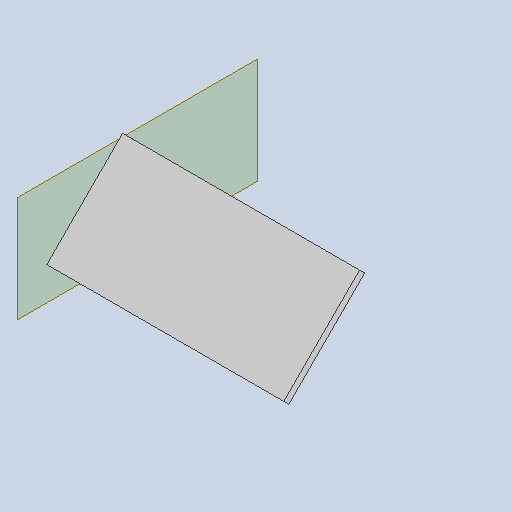
# Autodesk Inventor part: plugg
Saved by Autodesk Inventor 2022 (Build 260153000, 153)
## iProperties
Created: 2022-12-25
Part Number: plugg
Material: Generic
Document SubType Name: Modeling
Designer: Kamil
Density: 1 g/cm^3
Appearance: Default
Author: Kamil
Autodesk Inventor part; units mm, degrees
ref_plane "YZ Plane" through (0, 0, 0) normal (1, 0, 0) x (0, 1, 0)
ref_plane "XZ Plane" through (0, 0, 0) normal (0, 1, 0) x (-1, 0, 0)
ref_plane "Work Plane1" through (89.5496, -22.0458, 63.3377) normal (-1, 0, 0) x (0, -1, 0)
sketch "Sketch1" plane through (89.5496, -22.0458, 63.3377) normal (-1, 0, 0) x (0, -1, 0)
  line L0 (17.6, -19.3036) -> (17.6, 37.9036) projected
  line L1 (17.6, 37.9036) -> (-22.6, -2.2964) projected
  line L2 (-22.6, -2.2964) -> (-22.6, -53.1036) projected
  line L3 (-22.6, -53.1036) -> (-14.1, -53.1036) projected
  line L4 (-14.1, -53.1036) -> (-14.1, -37.9036) projected
  arc A0 (4.5, -19.3036) -> (-14.1, -37.9036) centre (4.5, -37.9036) ccw projected
  line L5 (4.5, -19.3036) -> (17.6, -19.3036) projected
  line L6 (20.6, 45.1462) -> (20.6, 40.9036) projected
  line L7 (5.7508, 30.297) -> (20.6, 45.1462) projected
  line L8 (7.8721, 28.1756) -> (5.7508, 30.297) projected
  line L9 (20.6, 40.9036) -> (7.8721, 28.1756) projected
  line L10 (7.8721, 28.1756) -> (6.4579, 29.5899)
  line L11 (6.4579, 29.5899) -> (-23.1664, -0.0344)
  line L12 (-22.6, -2.2964) -> (-23.795, -3.4915)
  line L13 (-23.795, -3.4915) -> (-26.5199, -0.7666)
  line L14 (-23.1664, -0.0344) -> (-26.5411, -3.4091)
  point P0 (-22.0458, -63.3377)
  point P1 (-25.2092, -2.0772)
  dimension "d0" = 2
  constraints: 10 end point, 3 perpendicular, 2 parallel, 1 point on line
  measures "d0" distance of L8.start L10.end
ref_plane "Work Plane2" through (188.5496, -39.6458, 10.2341) normal (1, 0, 0) x (0, 1, 0)
extrude "Extrusion1" add sketch "Sketch1" against normal up to surface (99 mm away) contours L1 L12 L13 L14 L11 L8
sketch "Sketch2" plane through (89.5496, 3.1634, 61.2604) normal (0, 0.7071, 0.7071) x (1, 0, 0)
  line L0 (99, -44.784) -> (99, 0) projected
  line L1 (0, 0) -> (99, 0) projected
  line L2 (0, -44.784) -> (0, 0) projected
  line L3 (0, -44.784) -> (99, -44.784) projected
  point P0 (-89.5496, 41.0808)
extrude "Extrusion2" add sketch "Sketch2" along normal blind 1
body "Solid1"
